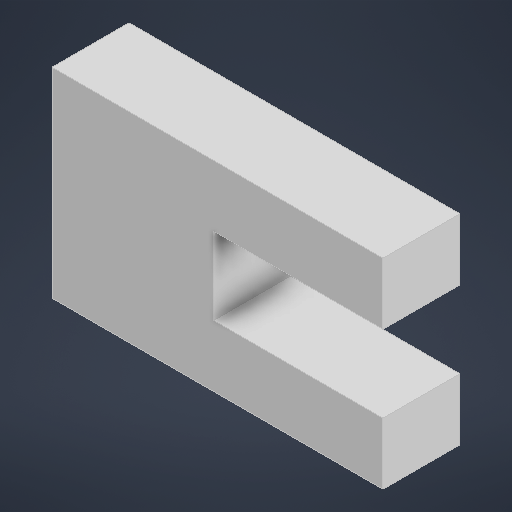
# Autodesk Inventor part: pitahaya5
Saved by Autodesk Inventor 2026.3 (Build 303398000, 398)
## iProperties
Created: 2024-05-08
Part Number: pitahaya5
Material: Generic
Document SubType Name: Modeling
Designer: Wilhelm
Density: 1 g/cm^3
Appearance: Default
Author: Wilhelm
Autodesk Inventor part; units mm, degrees
ref_plane "YZ Plane" through (0, 0, 0) normal (1, 0, 0) x (0, 1, 0)
ref_plane "XZ Plane" through (0, 0, 0) normal (0, 1, 0) x (-1, 0, 0)
ref_plane "XY Plane" through (0, 0, 0) normal (0, 0, 1) x (1, 0, 0)
sketch "Sketch1" plane through (0, 0, 0) normal (0, 0, 1) x (1, 0, 0)
  line L0 (5.375, 3.25) -> (5.375, 1.25)
  line L1 (5.375, 1.25) -> (-0.125, 1.25)
  line L2 (-0.125, 1.25) -> (-0.125, -1.25)
  line L3 (-0.125, -1.25) -> (5.375, -1.25)
  line L4 (5.375, -1.25) -> (5.375, -3.25)
  line L5 (5.375, -3.25) -> (-5.375, -3.25)
  line L6 (-5.375, -3.25) -> (-5.375, 3.25)
  line L7 (-5.375, 3.25) -> (5.375, 3.25)
  line L8 (-12.6672, 0) -> (12.6672, 0) construction
  line L9 (0, 8.1446) -> (0, -8.1446) construction
  point P0 (0, 0)
  point P1 (0, 0)
  dimension "d1" = 6.5
  dimension "d2" = 10.75
  dimension "d4" = 2.5
  dimension "d7" = 0.125
  constraints: 20 end point, 6 perpendicular, 2 midpoint, 2 point on line, 2 vertical, 1 coincident, 1 horizontal, 3 other
  measures "d1" distance of L5.end L6.end
  measures "d2" distance of L6.end L0.start
  measures "d4" distance between parallel lines of L3 L1
  measures "d7" distance between parallel lines of L9 L2
extrude "Extrusion1" add sketch "Sketch1" along normal mid plane 2.5
body "Solid1"
